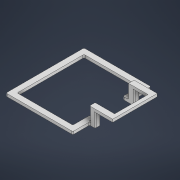
# Autodesk Inventor part: DrzakLEDky
Saved by Autodesk Inventor 2022 (Build 260153000, 153)
## iProperties
Created: 2023-04-13
Part Number: DrzakLEDky
Material: Všeobecné
Document SubType Name: Modeling
Designer: tada
Density: 1 g/cm^3
Appearance: Výchozí
Author: tada
Autodesk Inventor part; units mm, degrees
ref_plane "YZ Plane" through (0, 0, 0) normal (1, 0, 0) x (0, 1, 0)
ref_plane "XZ Plane" through (0, 0, 0) normal (0, 1, 0) x (-1, 0, 0)
ref_plane "XY Plane" through (0, 0, 0) normal (0, 0, 1) x (1, 0, 0)
sketch "Náčrt1" plane through (0, 0, 0) normal (0, 1, 0) x (-1, 0, 0)
  line L0 (50, 60) -> (-50, 60)
  line L1 (-50, 60) -> (-50, -60)
  line L2 (-50, -60) -> (50, -60)
  line L3 (50, -60) -> (50, 60)
  line L4 (60, 70) -> (-60, 70)
  line L5 (-60, 70) -> (-60, -70)
  line L6 (-60, -70) -> (60, -70)
  line L7 (60, -70) -> (60, 70)
  point P0 (0, 0)
  dimension "d1" = 100
  dimension "d2" = 120
  dimension "d3" = 10
  dimension "d4" = 10
  dimension "d5" = 10
  dimension "d6" = 10
  dimension "d9" = 60
  dimension "d10" = 50
  constraints: 16 end point, 4 parallel, 2 horizontal, 2 perpendicular
  measures "d1" distance of L0.start L0.end
  measures "d2" distance of L2.end L0.start
  measures "d3" distance between parallel lines of L7 L3
  measures "d4" distance between parallel lines of L4 L0
  measures "d5" distance between parallel lines of L6 L2
  measures "d6" distance between parallel lines of L1 L5
  measures "d9" distance from line of L0 point (0, 0)
  measures "d10" distance from line of L3 point (0, 0)
extrude "Vysunutí1" add sketch "Náčrt1" along normal blind 5
sketch "Náčrt3" plane through (60, 0, 70) normal (1, 0, 0) x (0, 0, -1)
  line L0 (10, 0) -> (130, 0) projected
  line L1 (30, 0) -> (40, 0)
  line L2 (40, 0) -> (40, 25)
  line L3 (40, 25) -> (30, 25)
  line L4 (30, 25) -> (30, 0)
  line L5 (100, 0) -> (110, 0)
  line L6 (110, 0) -> (110, 25)
  line L7 (110, 25) -> (100, 25)
  line L8 (100, 25) -> (100, 0)
  line L9 (140, 0) -> (140, 5) projected
  line L10 (0, 0) -> (0, 5) projected
  point P0 (70, 0)
  dimension "d35" = 25
  dimension "d36" = 25
  dimension "d37" = 10
  dimension "d38" = 10
  dimension "d39" = 60
  dimension "d40" = 30
  dimension "d41" = 30
  constraints: 16 end point, 4 parallel, 2 horizontal, 2 perpendicular, 2 point on line
  measures "d35" distance of L5.end L6.end
  measures "d36" distance of L3.end L1.start
  measures "d37" distance of L2.end L3.end
  measures "d38" distance of L6.end L7.end
  measures "d39" distance between parallel lines of L2 L8
  measures "d40" distance between parallel lines of L9 L6
  measures "d41" distance between parallel lines of L10 L4
extrude "Vysunutí3" add sketch "Náčrt3" along normal blind 10
sketch "Náčrt4" plane through (70, 0, 70) normal (1, 0, 0) x (0, 0, -1)
  line L0 (40, 25) -> (30, 25) projected
  line L1 (30, 25) -> (40, 25)
  line L2 (40, 25) -> (40, 30)
  line L3 (40, 30) -> (30, 30)
  line L4 (30, 30) -> (30, 25)
  line L5 (100, 25) -> (100, 0) projected
  line L6 (100, 25) -> (110, 25)
  line L7 (110, 25) -> (110, 30)
  line L8 (110, 30) -> (100, 30)
  line L9 (100, 30) -> (100, 25)
  point P0 (70, 0)
  dimension "d44" = 5
  dimension "d45" = 10
  dimension "d46" = 10
  dimension "d47" = 5
  constraints: 16 end point, 4 parallel, 2 horizontal, 2 perpendicular
  measures "d44" distance of L6.end L7.end
  measures "d45" distance of L7.end L8.end
  measures "d46" distance of L2.end L3.end
  measures "d47" distance of L1.end L2.end
extrude "Vysunutí4" add sketch "Náčrt4" along normal blind 25 and the other way blind 10
sketch "Náčrt5" plane through (95, 0, 70) normal (1, 0, 0) x (0, 0, -1)
  line L0 (40, 30) -> (30, 30) projected
  line L1 (110, 0) -> (110, 25) projected
  line L2 (30, 30) -> (110, 30)
  line L3 (110, 30) -> (110, 25)
  line L4 (110, 25) -> (30, 25)
  line L5 (30, 25) -> (30, 30)
  point P0 (70, 0)
  constraints: 8 end point, 2 parallel, 1 horizontal, 1 perpendicular
extrude "Vysunutí5" add sketch "Náčrt5" along normal blind 6.55
sketch "Náčrt6" plane through (0, 5, 0) normal (0, 1, 0) x (1, 0, 0)
  line L0 (60, -30) -> (70, -30) projected
  line L1 (50, 60) -> (50, -60) projected
  line L2 (60, -30) -> (50, -30)
  line L3 (50, -30) -> (50, 30)
  line L4 (50, 30) -> (60, 30)
  line L5 (60, 30) -> (60, -30)
  point P0 (0, 0)
  constraints: 8 end point, 2 parallel, 2 point on line, 1 horizontal, 1 perpendicular
extrude "Vysunutí6" cut sketch "Náčrt6" against normal blind 6.55
fillet "Zaoblení1" radius 2 8 edges at (50, 2.5, 60) (50, 2.5, -60) (-50, 2.5, -60) (-50, 2.5, 60) (-60, 2.5, 70) (60, 2.5, 70) (-60, 2.5, -70) (60, 2.5, -70)
fillet "Zaoblení2" radius 2 6 edges at (60, 2.5, -40) (70, 12.5, -40) (70, 12.5, -30) (70, 12.5, 30) (70, 12.5, 40) (60, 2.5, 40)
fillet "Zaoblení3" radius 2 4 edges at (60, 5, -35) (60, 5, 35) (60, 17.5, -40) (60, 17.5, 40)
fillet "Zaoblení4" radius 2 2 edges at (50, 2.5, -30) (50, 2.5, 30)
